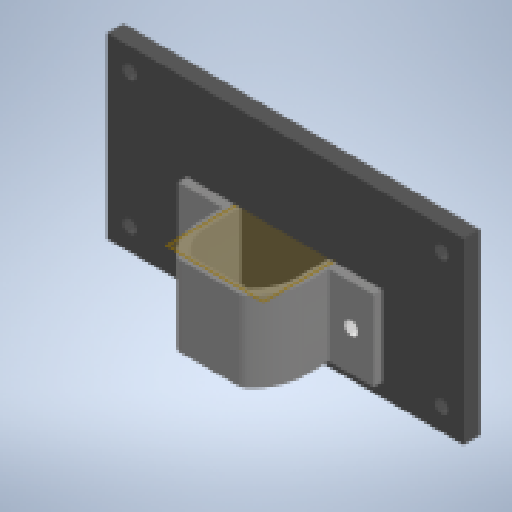
# Autodesk Inventor part: suporte_motor_1
Saved by Autodesk Inventor 2023 (Build 270158000, 158)
## iProperties
Created: 2022-09-27
Part Number: suporte_motor_1
Material: Generic
Document SubType Name: Modeling
Designer: kleber
Density: 1 g/cm^3
Appearance: Default
Author: kleber
Autodesk Inventor part; units mm, degrees
ref_plane "YZ Plane" through (0, 0, 0) normal (1, 0, 0) x (0, 1, 0)
ref_plane "XZ Plane" through (0, 0, 0) normal (0, 1, 0) x (-1, 0, 0)
ref_plane "XY Plane" through (0, 0, 0) normal (0, 0, 1) x (1, 0, 0)
sketch "Sketch1" plane through (0, 0, 0) normal (0, 0, 1) x (1, 0, 0)
  line L0 (-200, 100) -> (200, 100) projected
  line L1 (-200, -100) -> (-200, 100) projected
  line L2 (200, -100) -> (-200, -100) projected
  line L3 (200, 100) -> (200, -100) projected
  line L4 (-121, -18.2) -> (-94.2029, -18.2) projected
  line L5 (-94.2029, -18.2) -> (188.9125, -18.2)
  line L6 (110, -18.2) -> (70, -18.2)
  line L7 (70, -18.2) -> (150, -18.2)
  line L8 (150, -18.2) -> (150, -58.2)
  line L9 (150, -58.2) -> (70, -58.2)
  line L10 (70, -58.2) -> (70, -18.2)
  line L11 (150, -58.2) -> (145, -58.2)
  circle A0 centre (145, -53.2) radius 1.5
  circle A1 centre (145, -23.2) radius 1.5
  circle A2 centre (75, -23.2) radius 1.5
  circle A3 centre (75, -53.2) radius 1.5
  point P0 (0, 0)
  dimension "d2" = 80
  dimension "d3" = 40
  dimension "d4" = 5
  constraints: 14 end point, 4 centre point, 3 point on line, 2 horizontal, 2 parallel, 1 perpendicular
  measures "d2" distance of L8.end L9.end
  measures "d3" distance of L7.end L8.end
  measures "d4" distance of L8.end L11.end
extrude "Extrusion1" add sketch "Sketch1" along normal blind 3.7 contours L5 L8 L9 L10
ref_plane "Work Plane1" through (109.8736, -37.15, 11.15) normal (0, 1, 0) x (-1, 0, 0)
sketch "Sketch2" plane through (109.8736, -37.15, 11.15) normal (0, 1, 0) x (-1, 0, 0)
  line L0 (3.756, 7.45) -> (-3.756, 7.45)
  arc A0 (-6.6658, 7.3197) -> (-9.9, 0) centre (0, 0) ccw
  arc A1 (9.9, 0) -> (6.6658, 7.3197) centre (0, 0) ccw
  arc A2 (6.6658, 7.3197) -> (6.3291, 7.45) centre (6.3291, 6.95) ccw
  arc A3 (-6.3291, 7.45) -> (-6.6658, 7.3197) centre (-6.3291, 6.95) ccw
  line L1 (-3.756, 7.45) -> (-6.3291, 7.45)
  line L2 (6.3291, 7.45) -> (3.756, 7.45)
  arc A4 (-6.3291, 9.45) -> (-8.0124, 8.7984) centre (-6.3291, 6.95) ccw
  line L3 (-6.3291, 9.45) -> (-3.756, 9.45)
  line L4 (-3.756, 9.45) -> (3.756, 9.45)
  line L5 (3.756, 9.45) -> (6.3291, 9.45)
  arc A5 (8.0124, 8.7984) -> (6.3291, 9.45) centre (6.3291, 6.95) ccw
  line L6 (-11.9, 0) -> (-11.9, -5.45)
  line L7 (39.8736, -7.45) -> (-40.1264, -7.45) projected
  line L8 (-11.9, -7.45) -> (-21.9, -7.45)
  line L9 (-21.9, -7.45) -> (-21.9, -5.45)
  line L10 (-21.9, -5.45) -> (-11.9, -5.45)
  line L11 (11.9, -7.45) -> (21.9, -7.45)
  line L12 (21.9, -7.45) -> (21.9, -5.45)
  line L13 (21.9, -5.45) -> (11.9, -5.45)
  line L14 (9.9, 0) -> (9.9, -7.45)
  line L15 (-9.9, 0) -> (-9.9, -7.45)
  arc A6 (-8.0124, 8.7984) -> (-11.9, 0) centre (0, 0) ccw
  arc A7 (11.9, 0) -> (8.0124, 8.7984) centre (0, 0) ccw
  line L16 (11.9, 0) -> (11.9, -5.45)
  line L17 (-21.9, -7.45) -> (21.9, -7.45)
  point P0 (109.8736, -11.15)
  point P1 (21.9, -7.45)
  point P2 (-21.9, -7.45)
  dimension "d21" = 10
  dimension "d22" = 2
  dimension "d23" = 10
  dimension "d24" = 2
  dimension "d26" = 2
  constraints: 34 end point, 16 point on circle, 8 centre point, 4 parallel, 4 point on line, 2 horizontal, 2 perpendicular, 2 vertical, 1 collinear, 4 other
  measures "d21" distance of L6.end L9.end
  measures "d22" distance of L8.end L9.end
  measures "d23" distance of L13.end L12.end
  measures "d24" distance of L12.end L11.end
  measures "d26" distance between parallel lines of L6 L15
extrude "Extrusion2" add sketch "Sketch2" against normal blind 18 contours L0 L1 A3 A0 L15 L7 L9 L10 L6 A6 A4 L3 L4 L5 A5 A7 L16 L13 L12 L14 A1 A2 L2
sketch "Sketch3" plane through (121.7736, -37.15, 5.7) normal (0, 0, 1) x (1, 0, 0)
  line L0 (10, -18) -> (0, -18) projected
  circle A0 centre (5, -9) radius 1.5
  line L1 (-33.8, -18) -> (-33.8, 0) projected
  line L2 (-33.8, -18) -> (-33.8, -9)
  circle A1 centre (-28.8, -9) radius 1.5
  point P0 (-121.7736, 37.15)
  constraints: 2 centre point, 2 end point, 1 midpoint
hole "Hole1" at (126.7736, -46.15, 5.7) at (92.9736, -46.15, 5.7) direction (0, 0, -1) diameter 3 end through all
body "Solid1"
